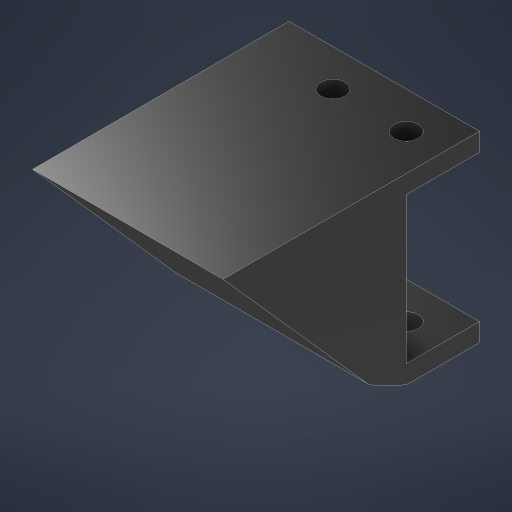
# Autodesk Inventor part: sleds v2 big
Saved by Autodesk Inventor 2024 (Build 280153000, 153)
## iProperties
Created: 2023-12-20
Part Number: sleds v2 big
Material: Generic
Document SubType Name: Modeling
Designer: elite
Density: 1 g/cm^3
Appearance: Glossy - Black
Author: elite
Autodesk Inventor part; units mm, degrees
ref_plane "YZ Plane" through (0, 0, 0) normal (1, 0, 0) x (0, 1, 0)
ref_plane "XZ Plane" through (0, 0, 0) normal (0, 1, 0) x (-1, 0, 0)
ref_plane "XY Plane" through (0, 0, 0) normal (0, 0, 1) x (1, 0, 0)
sketch "Sketch1" plane through (0, 0, 0) normal (1, 0, 0) x (0, 1, 0)
  line L0 (0, 0) -> (25.4, 0)
  line L1 (25.4, 0) -> (28.575, 0)
  line L2 (28.575, 0) -> (28.575, -12.7)
  line L3 (28.575, -12.7) -> (25.4, -12.7)
  line L4 (25.4, -12.7) -> (25.4, 0)
  line L5 (28.575, 0) -> (28.575, 31.75)
  line L6 (0, 0) -> (0, 6.35)
  line L7 (0, 6.35) -> (28.575, 31.75)
  line L8 (0, 0) -> (-3.175, 0)
  line L9 (-3.175, 0) -> (-3.175, -12.7)
  line L10 (-3.175, -12.7) -> (0, -12.7)
  line L11 (0, -12.7) -> (0, 0)
  line L12 (0, 6.35) -> (-3.175, 0)
  dimension "d0" = 25.4
  dimension "d1" = 3.175
  dimension "d2" = 12.7
  dimension "d3" = 31.75
  dimension "d16" = 6.35
  dimension "d17" = 3.175
  constraints: 26 end point, 6 perpendicular, 4 point on line, 1 horizontal, 1 vertical
  measures "d0" distance of L0.start L0.end
  measures "d1" distance of L0.end L1.end
  measures "d2" distance of L1.end L2.end
  measures "d3" distance of L1.end L5.end
  measures "d16" distance of L0.start L6.end
  measures "d17" distance of L0.start L8.end
extrude "Extrusion1" add sketch "Sketch1" along normal blind 53.34
sketch "Sketch2" plane through (0, 28.575, 31.75) normal (0, 1, 0) x (1, 0, 0)
  line L0 (53.34, 44.45) -> (53.34, 38.1)
  line L1 (53.34, 44.45) -> (53.34, 0) projected
  line L2 (53.34, 38.1) -> (26.67, 38.1)
  circle A0 centre (26.67, 38.1) radius 2.1082
  point P0 (0, 31.75)
  dimension "d6" = 6.35
  dimension "d7" = 26.67
  dimension "d8" = 4.2164
  constraints: 4 end point, 1 centre point, 1 coincident, 1 horizontal, 1 point on line
  measures "d6" distance of L0.start L0.end
  measures "d7" distance of L0.end L2.end
  measures "d8" diameter of A0
extrude "Extrusion2" cut sketch "Sketch2" against normal blind 43.815
sketch "Sketch3" plane through (53.34, 0, 0) normal (1, 0, 0) x (0, 0, -1)
  line L0 (12.7, 25.4) -> (12.7, 28.575) projected
  line L1 (12.7, 28.575) -> (-16.4619, 28.575)
  line L2 (-16.4619, 28.575) -> (-16.4619, 0)
  line L3 (-16.4619, 0) -> (12.7, 0)
  line L4 (12.7, 0) -> (12.7, 28.575)
  line L5 (-16.4619, 0) -> (-35.4962, 0)
  line L6 (-35.4962, 0) -> (-35.4962, 28.575)
  line L7 (-35.4962, 28.575) -> (-16.4619, 28.575)
  line L8 (-16.4619, 28.575) -> (-16.4619, 0)
  line L9 (12.7, -3.175) -> (12.7, 0) projected
  line L10 (12.7, 0) -> (-7.1998, 0)
  line L11 (-7.1998, 0) -> (-7.1998, -5.5168)
  line L12 (-7.1998, -5.5168) -> (12.7, -5.5168)
  line L13 (12.7, -5.5168) -> (12.7, 0)
  point P0 (0, 0)
  point P1 (12.7, 25.4)
  constraints: 24 end point, 6 parallel, 3 horizontal, 3 perpendicular
extrude "Extrusion3" cut sketch "Sketch3" against normal blind 20.32
sketch "Sketch4" plane through (0, 28.575, 31.75) normal (0, 1, 0) x (1, 0, 0)
  circle A0 centre (26.67, 38.1) radius 2.1082 projected
  line L0 (26.67, 38.1) -> (13.97, 38.1)
  circle A1 centre (13.97, 38.1) radius 2.1082
  point P0 (0, 31.75)
  dimension "d13" = 12.7
  constraints: 2 end point, 1 centre point, 1 coincident, 1 horizontal
  measures "d13" distance of L0.start L0.end
extrude "Extrusion4" cut sketch "Sketch4" against normal blind 2514.6 contours A1
fillet "Fillet1" radius 3.175 2 edges at (16.51, 0, 6.35) (16.51, -3.175, 0)
body "Solid1"
